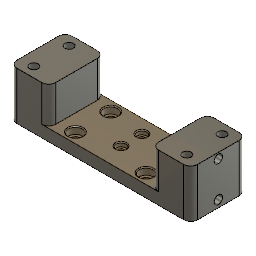
flexMount_v23 (Autodesk Fusion 360 design; units mm, degrees)
Autodesk Fusion 360 part; units mm, degrees
sketch "Sketch1" plane through (0, 0, 0) normal (0, 1, 0) x (1, 0, 0)
mesh "Mesh1" [no effect]
sketch "Sketch2" plane through (0, 0, 0) normal (0, 1, 0) x (1, 0, 0)
  line L0 (65, 20) -> (-65, 20)
  line L1 (-65, 20) -> (-65, -20)
  line L2 (-65, -20) -> (65, -20)
  line L3 (65, -20) -> (65, 20)
  line L4 (65, 20) -> (-65, -20) construction
  line L5 (-65, 20) -> (65, -20) construction
  dimension "d3" = 130
  dimension "d4" = 40
extrude "Extrude1" add sketch "Sketch2" along normal blind 6.6 makes body 1
sketch "Sketch4" plane through (0, 6.6, 0) normal (0, 1, 0) x (-1, 0, 0)
  line L0 (-65, 20) -> (-65, -20)
  line L1 (-65, -20) -> (65, -20)
  line L2 (65, -20) -> (65, 20)
  line L3 (65, 20) -> (-65, 20)
  line L4 (65, -20) -> (37, -20)
  line L5 (37, -20) -> (37, 20)
  line L6 (37, 20) -> (65, 20)
  line L7 (65, 20) -> (65, -20)
  dimension "d7" = 40
  dimension "d8" = 28
  measures "d7" distance of origin
sketch "Sketch5" plane through (0, 0, 0) normal (0, 0, 1) x (1, 0, 0)
extrude "Extrude2" add sketch "Sketch4" along normal blind 28 contours L1 L2 L3 L4 L5 L6 L7 bodies 1
sketch "Sketch6" plane through (0, 6.6, 0) normal (0, 1, 0) x (-1, 0, 0)
  line L0 (37, -20) -> (37, 20)
  line L1 (37, 20) -> (-65, 20)
  line L2 (-65, 20) -> (-65, -20)
  line L3 (-65, -20) -> (37, -20)
  line L4 (-65, -20) -> (-35, -20)
  line L5 (-35, -20) -> (-35, 20)
  line L6 (-35, 20) -> (-65, 20)
  line L7 (-65, 20) -> (-65, -20)
  dimension "d11" = 30
  dimension "d12" = 40
  measures "d12" distance of origin
extrude "Extrude3" add sketch "Sketch6" along normal blind 28 contours L1 L2 L3 L4 L5 L6 L7 bodies 1
hole "Hole1" at (-55, 34.6, -12.7) direction (0, -1, 0) diameter 6.1 depth 34.6 tip angle 180 bodies 1
hole "Hole2" at (-55, 34.6, 12.7) direction (0, -1, 0) diameter 6.1 depth 34.6 tip angle 180 bodies 1
hole "Hole3" at (55, 34.6, -12.7) direction (0, -1, 0) diameter 6.1 depth 34.6 tip angle 180 bodies 1
hole "Hole4" at (55, 34.6, 12.7) direction (0, -1, 0) diameter 6.1 depth 34.6 tip angle 180 bodies 1
fillet "Fillet1" radius 5 4 edges at (-37, 20.6, 20) (-37, 20.6, -20) (35, 20.6, 20) (65, 17.3, 20) on bodies 1
fillet "Fillet2" radius 5 2 edges at (-65, 17.3, -20) (-65, 17.3, 20) on bodies 1
fillet "Fillet3" radius 5 2 edges at (35, 20.6, -20) (65, 17.3, -20) on bodies 1
sketch "Sketch7" plane through (0, 0, 0) normal (0, 1, 0) x (1, 0, 0)
sketch "Sketch8" plane through (0, 0, 0) normal (0, 1, 0) x (1, 0, 0)
sketch "Sketch9" plane through (0, 0, 0) normal (0, 1, 0) x (1, 0, 0)
sketch "Sketch10" plane through (0, 0, 0) normal (0, 1, 0) x (1, 0, 0)
sketch "Sketch11" plane through (0, 0, 0) normal (0, -1, 0) x (1, 0, 0)
  arc A0 (60, -20) -> (65, -15) centre (60, -15) ccw
  line L0 (65, -15) -> (65, 15)
  arc A1 (65, 15) -> (60, 20) centre (60, 15) ccw
  line L1 (60, 20) -> (-60, 20)
  arc A2 (-60, 20) -> (-65, 15) centre (-60, 15) ccw
  line L2 (-65, 15) -> (-65, -15)
  arc A3 (-65, -15) -> (-60, -20) centre (-60, -15) ccw
  line L3 (-60, -20) -> (60, -20)
  circle A4 centre (-55, -12.7) radius 3.05
  circle A5 centre (-55, 12.7) radius 3.05
  circle A6 centre (55, -12.7) radius 3.05
  circle A7 centre (55, 12.7) radius 3.05
  line L4 (0, 0) -> (0, -50)
  line L5 (0, -20) -> (-6.35, -20)
  line L6 (-6.35, -20) -> (6.35, -20)
  line L7 (6.35, -20) -> (6.35, 6)
  line L8 (6.35, 6) -> (-6.35, 6)
  line L9 (-6.35, 6) -> (-6.35, -20)
  dimension "d38" = 6.35
  dimension "d39" = 12.7
  dimension "d40" = 26
sketch "Sketch12" plane through (0, 0, 0) normal (1, 0, 0) x (0, 0, -1)
extrude "Extrude4" cut sketch "Sketch11" against normal blind 0.6 contours L3 L5 L6 L7 L8 L9 bodies 1
extrude "Extrude5" add 1 faces at (-21.5755, 0, -8.6738) along direction (0, -1, 0) blind 2 on bodies 1 bodies 1
hole "Hole5" at (0, 34.6, -10) direction (0, -1, 0) diameter 3.9 depth 46 tip angle 180 bodies 1
sketch "Sketch13" plane through (0, -2, 0) normal (0, -1, 0) x (1, 0, 0)
  circle A0 centre (55, 12.7) radius 3.05
  circle A1 centre (55, -12.7) radius 3.05
  circle A2 centre (-55, 12.7) radius 3.05
  circle A3 centre (-55, -12.7) radius 3.05
  line L0 (-6.35, -20) -> (-6.35, 6)
  line L1 (-6.35, 6) -> (6.35, 6)
  line L2 (6.35, 6) -> (6.35, -20)
  line L3 (6.35, -20) -> (60, -20)
  arc A4 (60, -20) -> (65, -15) centre (60, -15) ccw
  line L4 (65, -15) -> (65, 15)
  arc A5 (65, 15) -> (60, 20) centre (60, 15) ccw
  line L5 (60, 20) -> (-60, 20)
  arc A6 (-60, 20) -> (-65, 15) centre (-60, 15) ccw
  line L6 (-65, 15) -> (-65, -15)
  arc A7 (-65, -15) -> (-60, -20) centre (-60, -15) ccw
  line L7 (-60, -20) -> (-6.35, -20)
  line L8 (-6.35, 6) -> (6.35, 6)
  line L9 (6.35, 6) -> (6.35, 15)
  line L10 (6.35, 15) -> (-6.35, 15)
  line L11 (-6.35, 15) -> (-6.35, 6)
  dimension "d50" = 9
extrude "Extrude6" cut sketch "Sketch13" against normal blind 2.6 contours L1 L8 L9 L10 L11 bodies 1
extrude "Extrude7" cut 1 faces at (0, 0.6, 7.3167) along direction (0, 1, 0) blind 1 on bodies 1 bodies 1
hole "Hole6" at (0, 6.6, 5) direction (0, -1, 0) diameter 3.9 depth 46 tip angle 180 bodies 1
hole "Hole7" at (0, 6.6, -10) direction (0, -1, 0) diameter 7 depth 3 tip angle 180 bodies 1
extrude "Extrude8" cut 1 faces at (0, 1.6, -17.3167) along direction (0, 1, 0) blind 1 on bodies 1 bodies 1
hole "Hole8" at (0, 6.6, 5) direction (0, -1, 0) diameter 7 depth 3 tip angle 180 bodies 1
fillet "Fillet4" radius 0.6 2 edges at (1.2657, 6.6, 1.7369) (1.2657, 6.6, -13.2631) on bodies 1
hole "Hole9" at (25.7, 6.6, -12.7) direction (0, -1, 0) diameter 10 depth 5 tip angle 180 bodies 1
hole "Hole10" at (-25.1, 6.6, -12.7) direction (0, -1, 0) diameter 10 depth 5 tip angle 180 bodies 1
hole "Hole11" at (25.7, 6.6, 12.7) direction (0, -1, 0) diameter 10 depth 5 tip angle 180 bodies 1
hole "Hole12" at (-25.1, 6.6, 12.7) direction (0, -1, 0) diameter 10 depth 5 tip angle 180 bodies 1
hole "Hole13" at (25.7, 1.6, -12.7) direction (0, -1, 0) diameter 6.1 depth 5 tip angle 180 bodies 1
hole "Hole14" at (25.7, 1.6, 12.7) direction (0, -1, 0) diameter 6.1 depth 5 tip angle 180 bodies 1
hole "Hole15" at (-25.1, 1.6, 12.7) direction (0, -1, 0) diameter 6.1 depth 5 tip angle 180 bodies 1
hole "Hole16" at (-25.1, 1.6, -12.7) direction (0, -1, 0) diameter 6.1 depth 5 tip angle 180 bodies 1
fillet "Fillet5" radius 0.6 4 edges at (-23.2919, 6.6, 8.0384) (27.5081, 6.6, 8.0384) (27.5081, 6.6, -17.3616) (-23.2919, 6.6, -17.3616) on bodies 1
hole "Hole17" at (-65, 29.6, 0) direction (1, 0, 0) diameter 6.1 depth 8 tip angle 180 bodies 1
hole "Hole18" at (-65, 4.2, 0) direction (1, 0, 0) diameter 6.1 depth 8 tip angle 180 bodies 1
hole "Hole19" at (65, 29.6, 0) direction (-1, 0, 0) diameter 6.1 depth 8 tip angle 180 bodies 1
hole "Hole20" at (65, 4.2, 0) direction (-1, 0, 0) diameter 6.1 depth 8 tip angle 180 bodies 1
delete_face "DeleteFace1" 1 faces at (39.7621, 15.9333, 19.9943) on bodies 1
delete_face "DeleteFace2" 1 faces at (35.0057, 15.9333, -15.2379) on bodies 1
sketch "Sketch14" plane through (0, 6.6, 0) normal (0, 1, 0) x (-1, 0, 0)
  line L0 (-35, 20) -> (-35, -20)
  line L1 (-35, -20) -> (42, -20)
  arc A0 (37, -15) -> (42, -20) centre (42, -15) ccw
  line L2 (37, -15) -> (37, 15)
  arc A1 (42, 20) -> (37, 15) centre (42, 15) ccw
  line L3 (42, 20) -> (-35, 20)
  circle A2 centre (-25.7, -12.7) radius 5.6
  circle A3 centre (25.1, 12.7) radius 5.6
  circle A4 centre (0, 5) radius 4.1
  circle A5 centre (0, -10) radius 4.1
  circle A6 centre (-25.7, 12.7) radius 5.6
  circle A7 centre (25.1, -12.7) radius 5.6
sketch "Sketch15" plane through (0, 34.6, 0) normal (0, 1, 0) x (-1, 0, 0)
  line L0 (-35, -20) -> (-35, 20)
  line L1 (-35, 20) -> (-60, 20)
  arc A0 (-60, 20) -> (-65, 15) centre (-60, 15) ccw
  line L2 (-65, 15) -> (-65, -15)
  arc A1 (-65, -15) -> (-60, -20) centre (-60, -15) ccw
  line L3 (-60, -20) -> (-35, -20)
  circle A2 centre (-55, 12.7) radius 3.05
  circle A3 centre (-55, -12.7) radius 3.05
  line L4 (-35, -20) -> (-37, -20)
  line L5 (-37, -20) -> (-37, 20)
  line L6 (-37, 20) -> (-35, 20)
  line L7 (-35, 20) -> (-35, -20)
  dimension "d122" = 2
  dimension "d123" = 40
  measures "d123" distance of origin
extrude "Extrude9" cut sketch "Sketch15" against normal blind 28 contours L0 L1 L3 L4 L5 L6 L7 bodies 1
fillet "Fillet6" radius 5 2 edges at (37, 20.6, -20) (37, 20.6, 20) on bodies 1
extrude "Extrude10" add 1 faces at (0, 2.6, -17.3167) along direction (0, -1, 0) blind 2 on bodies 1 bodies 1
delete_face "DeleteFace3" 1 faces at (-59.6667, 29.9037, 3.0348) on bodies 1
delete_face "DeleteFace4" 1 faces at (-59.6667, 4.5037, 3.0348) on bodies 1
delete_face "DeleteFace5" 1 faces at (59.6667, 29.9037, -3.0348) on bodies 1
delete_face "DeleteFace6" 1 faces at (59.6667, 4.5037, -3.0348) on bodies 1
sketch "Sketch16" plane through (0, -2, 0) normal (0, -1, 0) x (1, 0, 0)
  circle A0 centre (-25.1, -12.7) radius 3.05
  circle A1 centre (-25.1, 12.7) radius 3.05
  circle A2 centre (25.7, 12.7) radius 3.05
  circle A3 centre (25.7, -12.7) radius 3.05
  line L0 (6.35, 15) -> (6.35, -20)
  line L1 (6.35, -20) -> (60, -20)
  arc A4 (60, -20) -> (65, -15) centre (60, -15) ccw
  line L2 (65, -15) -> (65, 15)
  arc A5 (65, 15) -> (60, 20) centre (60, 15) ccw
  line L3 (60, 20) -> (-60, 20)
  arc A6 (-60, 20) -> (-65, 15) centre (-60, 15) ccw
  line L4 (-65, 15) -> (-65, -15)
  arc A7 (-65, -15) -> (-60, -20) centre (-60, -15) ccw
  line L5 (-60, -20) -> (-6.35, -20)
  line L6 (-6.35, -20) -> (-6.35, 15)
  line L7 (-6.35, 15) -> (6.35, 15)
  circle A8 centre (55, 12.7) radius 3.05
  circle A9 centre (55, -12.7) radius 3.05
  circle A10 centre (-55, 12.7) radius 3.05
  circle A11 centre (-55, -12.7) radius 3.05
  line L8 (-4.889, -20) -> (5.511, -20)
  line L9 (5.511, -20) -> (5.511, 14)
  line L10 (5.511, 14) -> (-4.889, 14)
  line L11 (-4.889, 14) -> (-4.889, -20)
  line L12 (-6.35, -20) -> (6.35, -20)
  dimension "d129" = 10.4
extrude "Extrude11" add sketch "Sketch16" against normal blind 2.2 separate body contours L8 L9 L10 L11 L12 makes body 2
sketch "Sketch17" plane through (0, -2, 0) normal (0, -1, 0) x (1, 0, 0)
  line L0 (-4.889, 14) -> (-4.889, -20)
  line L1 (-4.889, -20) -> (5.511, -20)
  line L2 (5.511, -20) -> (5.511, 14)
  line L3 (5.511, 14) -> (-4.889, 14)
  line L4 (-1, 14) -> (0, 14)
  line L5 (0, 14) -> (0, 15)
  line L6 (0, 15) -> (-1, 15)
  line L7 (-1, 15) -> (-1, 14)
  line L8 (-6.35, 15) -> (6.35, 15)
extrude "Extrude12" add sketch "Sketch17" against normal blind 2.4 contours L3 L4 L5 L6 L7 L8 bodies 1 2
extrude "Extrude13" cut 2 faces at (42.2936, 34.6, 3.5022) (-42.2936, 34.6, 3.5022) along direction (0, -1, 0) blind 2 on bodies 1 bodies 1
hole "Hole21" at (65, 28.6, 0) direction (-1, 0, 0) diameter 6.1 depth 8 tip angle 180 bodies 1
hole "Hole22" at (65, 3.2, 0) direction (-1, 0, 0) diameter 6.1 depth 8 tip angle 180 bodies 1
hole "Hole23" at (-65, 28.6, 0) direction (1, 0, 0) diameter 6.1 depth 8 tip angle 180 bodies 1
hole "Hole24" at (-65, 3.2, 0) direction (1, 0, 0) diameter 6.1 depth 8 tip angle 180 bodies 1
